Autodesk Fusion 360 part; units mm, degrees
note: some values were not read from the file. Set by a fixed rule: which sketch regions a step uses.
(part 2 of 4)
  spline S109 degree 3 poles (-112.0728, -32.2292) (-112.5404, -31.8601) (-113.2203, -31.6275) (-113.5837, -31.7122) knots 0 0 0 0 1 1 1 1
  spline S110 degree 3 poles (-136.2209, -38.6484) (-139.7578, -43.5067) (-144.003, -49.2146) (-147.0742, -52.9444) knots 0 0 0 0 1 1 1 1
  spline S111 degree 3 poles (-154.2165, -27.0184) (-154.4007, -27.683) (-154.551, -27.4601) (-154.6666, -26.3504) knots 0 0 0 0 1 1 1 1
  spline S112 degree 3 poles (-84.3741, -40.3079) (-87.8752, -40.018) (-88.8355, -39.1456) (-87.7319, -37.2577) knots 0 0 0 0 1 1 1 1
  spline S113 degree 3 poles (-140.3165, -99.6255) (-140.307, -99.0782) (-141.0618, -97.9071) (-141.9939, -97.0229) knots 0 0 0 0 1 1 1 1
  line L97 (-121.5387, -89.9657) -> (-118.5791, -90.609)
  spline S114 degree 3 poles (-154.7919, -33.624) (-155.1377, -31.5295) (-154.9908, -31.2048) (-153.5956, -30.9793) knots 0 0 0 0 1 1 1 1
  spline S115 degree 3 poles (-103.6508, -80.373) (-104.0694, -84.1491) (-102.7518, -86.3818) (-98.6044, -88.9248) knots 0 0 0 0 1 1 1 1
  spline S116 degree 3 poles (-104.4545, -159.4656) (-104.6393, -158.9576) (-105.2292, -158.3375) (-105.7651, -158.0876) knots 0 0 0 0 1 1 1 1
  line L98 (-76.19, -217.0111) -> (-79.4365, -211.2784)
  spline S117 degree 3 poles (-96.7029, -170.3232) (-100.0171, -162.0462) (-100.2006, -161.7333) (-102.1257, -161.073) knots 0 0 0 0 1 1 1 1
  spline S118 degree 3 poles (-106.4868, -123.3433) (-106.9706, -124.7012) (-107.6243, -126.5592) (-107.9395, -127.4722) knots 0 0 0 0 1 1 1 1
  line L99 (-151.1746, -82.8005) -> (-152.1113, -79.6578)
  spline S119 degree 3 poles (-164.6222, -35.8254) (-164.3798, -35.5183) (-164.0173, -35.7185) (-163.8165, -36.2701) knots 0 0 0 0 1 1 1 1
  spline S120 degree 3 poles (-97.3886, -94.7063) (-100.0855, -99.9855) (-102.1641, -106.0488) (-104.0281, -114.0757) knots 0 0 0 0 1 1 1 1
  spline S121 degree 3 poles (-116.5906, -88.5651) (-114.2332, -86.142) (-111.3799, -79.5261) (-109.9199, -73.0985) knots 0 0 0 0 1 1 1 1
  line L100 (-71.6837, -54.5973) -> (-71.6834, -54.5969)
  spline S122 degree 3 poles (-119.4232, -30.4738) (-125.5719, -30.4722) (-132.2129, -34.4961) (-136.2209, -38.6484) knots 0 0 0 0 1 1 1 1
  spline S123 degree 3 poles (-87.3826, -35.3672) (-87.8899, -33.9734) (-86.4389, -25.012) (-85.4231, -23.2654) knots 0 0 0 0 1 1 1 1
  spline S124 degree 3 poles (-154.6666, -26.3504) (-155.4003, -19.3112) (-156.3482, -18.6133) (-162.7786, -20.375) knots 0 0 0 0 1 1 1 1
  spline S125 degree 3 poles (-109.9199, -73.0985) (-108.891, -68.5684) (-108.2546, -67.383) (-107.6608, -68.8907) knots 0 0 0 0 1 1 1 1
  spline S126 degree 3 poles (-83.0888, -107.0535) (-83.9086, -107.766) (-83.3399, -110.3472) (-82.4356, -110.0181) knots 0 0 0 0 1 1 1 1
  spline S127 degree 3 poles (-145.3026, -92.1497) (-146.1903, -90.3535) (-147.6639, -88.2222) (-148.5772, -87.4136) knots 0 0 0 0 1 1 1 1
  line L101 (-127.616, -73.2152) -> (-127.616, -73.215)
  spline S128 degree 3 poles (-179.1592, -14.8194) (-179.6701, -15.4667) (-181.8024, -11.7834) (-183.7113, -6.9562) knots 0 0 0 0 1 1 1 1
  spline S129 degree 3 poles (-162.4907, -49.7556) (-162.586, -51.9164) (-162.5668, -52.4177) (-162.3525, -53.3552) knots 0 0 0 0 1 1 1 1
  spline S130 degree 3 poles (-108.3458, -30.6552) (-107.7548, -30.7777) (-107.7164, -30.5518) (-108.2282, -29.9629) knots 0 0 0 0 1 1 1 1
  spline S131 degree 3 poles (-107.3197, -33.1494) (-108.6187, -32.1334) (-109.3089, -30.4554) (-108.3458, -30.6552) knots 0 0 0 0 1 1 1 1
  spline S132 degree 3 poles (-130.5025, -128.6131) (-135.3605, -121.8502) (-135.4133, -121.7401) (-135.9917, -117.1824) knots 0 0 0 0 1 1 1 1
  spline S133 degree 3 poles (-82.4356, -110.0181) (-81.5449, -109.6939) (-77.0276, -113.218) (-76.5096, -114.6411) knots 0 0 0 0 1 1 1 1
  spline S134 degree 3 poles (-126.1453, -138.8187) (-126.7195, -138.8087) (-127.4424, -138.105) (-127.7519, -137.2548) knots 0 0 0 0 1 1 1 1
  spline S135 degree 3 poles (-139.0681, -102.1478) (-138.9659, -101.4044) (-139.1827, -100.8591) (-139.6164, -100.7692) knots 0 0 0 0 1 1 1 1
  line L102 (-95.4296, -90.8714) -> (-97.3886, -94.7063)
  spline S136 degree 3 poles (-108.2282, -29.9629) (-108.6756, -29.448) (-108.6885, -28.9597) (-108.2594, -28.7749) knots 0 0 0 0 1 1 1 1
  spline S137 degree 3 poles (-115.0249, -149.0253) (-116.7184, -147.2776) (-118.5469, -145.7771) (-120.0633, -144.8906) knots 0 0 0 0 1 1 1 1
  line L103 (-152.1113, -79.6578) -> (-148.5919, -78.2652)
  spline S138 degree 3 poles (-124.7918, -139.6875) (-124.9621, -139.2197) (-125.5712, -138.8287) (-126.1453, -138.8187) knots 0 0 0 0 1 1 1 1
  line L104 (-148.5919, -78.2652) -> (-145.0725, -76.8727)
  spline S139 degree 3 poles (-74.1947, -115.3174) (-73.0292, -114.8932) (-71.9308, -114.9941) (-71.1607, -115.5962) knots 0 0 0 0 1 1 1 1
  spline S140 degree 3 poles (-129.6791, -65.9357) (-125.8343, -62.6694) (-127.4522, -73.1016) (-127.616, -73.2152) knots 0 0 0 0 1 1 1 1
  spline S141 degree 3 poles (-93.212, -111.5023) (-91.5685, -106.4875) (-88.2032, -100.9795) (-84.6693, -97.5197) knots 0 0 0 0 1 1 1 1
  spline S142 degree 3 poles (-127.616, -73.215) (-127.919, -73.3253) (-128.2661, -73.1431) (-128.3872, -72.8102) knots 0 0 0 0 1 1 1 1
  spline S143 degree 3 poles (-137.8943, -108.0755) (-138.633, -105.4917) (-139.1612, -102.8242) (-139.0681, -102.1478) knots 0 0 0 0 1 1 1 1
  spline S144 degree 3 poles (-85.4231, -23.2654) (-84.2448, -21.2393) (-84.8036, -21.3276) (-87.2116, -23.5478) knots 0 0 0 0 1 1 1 1
  spline S145 degree 3 poles (-127.7519, -137.2548) (-128.1329, -136.2081) (-128.6652, -135.819) (-129.4007, -136.0498) knots 0 0 0 0 1 1 1 1
  spline S146 degree 3 poles (-133.2081, -68.992) (-131.2389, -68.4482) (-130.936, -67.0047) (-129.6791, -65.9357) knots 0 0 0 0 1 1 1 1
  spline S147 degree 3 poles (-183.7113, -6.9562) (-184.7798, -4.2542) (-185.4511, -3.3311) (-186.5872, -3.0015) knots 0 0 0 0 1 1 1 1
  spline S148 degree 3 poles (-103.4783, -30.4373) (-102.821, -31.518) (-102.6423, -32.3115) (-103.0249, -32.4507) knots 0 0 0 0 1 1 1 1
  line L105 (-118.5791, -90.609) -> (-116.5906, -88.5651)
  spline S149 degree 3 poles (-107.6608, -68.8907) (-107.497, -69.3066) (-106.4548, -71.4025) (-105.3449, -73.5484) knots 0 0 0 0 1 1 1 1
  spline S150 degree 3 poles (-103.1195, -33.1042) (-102.17, -33.8536) (-103.886, -34.7192) (-105.7404, -34.4262) knots 0 0 0 0 1 1 1 1
  spline S151 degree 3 poles (-165.6722, -35.9026) (-165.337, -36.1672) (-164.8645, -36.1324) (-164.6222, -35.8254) knots 0 0 0 0 1 1 1 1
  spline S152 degree 3 poles (-84.6693, -97.5197) (-83.6282, -96.5006) (-82.5684, -95.831) (-82.3142, -96.0317) knots 0 0 0 0 1 1 1 1
  spline S153 degree 3 poles (-148.5772, -87.4136) (-149.6517, -86.4623) (-150.5685, -84.8339) (-151.1746, -82.8005) knots 0 0 0 0 1 1 1 1
  spline S154 degree 3 poles (-104.0281, -114.0757) (-104.8966, -117.815) (-106.003, -121.9853) (-106.4868, -123.3433) knots 0 0 0 0 1 1 1 1
  spline S155 degree 3 poles (-95.9356, -117.5951) (-95.3387, -116.9936) (-94.113, -114.2518) (-93.212, -111.5023) knots 0 0 0 0 1 1 1 1
  spline S156 degree 3 poles (-165.5322, -47.9185) (-167.9275, -39.8001) (-167.9943, -34.07) (-165.6722, -35.9025) knots 0 0 0 0 1 1 1 1
  line L106 (-139.6588, -79.8807) -> (-139.6591, -79.8813)
  spline S157 degree 3 poles (-163.8165, -36.2701) (-163.3332, -37.5981) (-162.3816, -47.2782) (-162.4907, -49.7556) knots 0 0 0 0 1 1 1 1
  spline S158 degree 3 poles (-99.4834, -22.2152) (-102.7671, -24.1219) (-105.1902, -27.5695) (-103.4783, -30.4373) knots 0 0 0 0 1 1 1 1
  spline S159 degree 3 poles (-70.9678, -64.1804) (-71.0778, -65.837) (-71.2409, -67.2189) (-71.3304, -67.2515) knots 0 0 0 0 1 1 1 1
  spline S160 degree 3 poles (-100.1317, -132.8949) (-98.7815, -129.5666) (-97.5292, -125.0086) (-97.3489, -122.7659) knots 0 0 0 0 1 1 1 1
  spline S161 degree 3 poles (-113.5837, -31.7122) (-114.8758, -31.1202) (-118.9006, -30.5) (-119.4232, -30.4738) knots 0 0 0 0 1 1 1 1
  spline S162 degree 3 poles (-71.3304, -67.2515) (-72.5816, -66.2567) (-96.5427, -51.7484) (-92.0911, -45.0244) knots 0 0 0 0 1 1 1 1
  spline S163 degree 3 poles (-105.3449, -73.5484) (-103.5984, -76.9253) (-103.3705, -77.8432) (-103.6508, -80.373) knots 0 0 0 0 1 1 1 1
  spline S164 degree 3 poles (-87.7319, -37.2577) (-87.3803, -36.6562) (-87.2231, -35.8055) (-87.3826, -35.3672) knots 0 0 0 0 1 1 1 1
  spline S165 degree 3 poles (-147.0742, -52.9444) (-148.0276, -54.2206) (-148.1757, -54.2339) (-148.9598, -53.1145) knots 0 0 0 0 1 1 1 1
  spline S166 degree 3 poles (-97.3489, -122.7659) (-97.1686, -120.5233) (-96.5325, -118.1966) (-95.9356, -117.5951) knots 0 0 0 0 1 1 1 1
  line L107 (122.5483, 261.5188) -> (122.5506, 261.5232)
  spline S167 degree 3 poles (-177.1846, -17.5625) (-177.5438, -16.9549) (-178.0397, -15.9683) (-178.2865, -15.3701) knots 0 0 0 0 1 1 1 1
  spline S168 degree 3 poles (-110.1669, -137.8907) (-112.712, -151.3653) (-112.7265, -151.3976) (-115.0249, -149.0253) knots 0 0 0 0 1 1 1 1
  spline S169 degree 3 poles (-139.6164, -100.7692) (-140.0109, -100.6874) (-140.326, -100.1727) (-140.3165, -99.6255) knots 0 0 0 0 1 1 1 1
  line L108 (-165.6722, -35.9025) -> (-165.6722, -35.9026)
  spline S170 degree 3 poles (-91.5548, -189.9237) (-92.8333, -186.2605) (-93.4883, -183.3011) (-93.4037, -181.5704) knots 0 0 0 0 1 1 1 1
  spline S171 degree 3 poles (-105.7404, -34.4262) (-106.729, -34.2701) (-107.319, -34.0516) (-107.0516, -33.9408) knots 0 0 0 0 1 1 1 1
  spline S172 degree 3 poles (-84.6389, -203.663) (-86.6971, -201.6816) (-90.5134, -195.9478) (-89.9214, -195.7261) knots 0 0 0 0 1 1 1 1
  spline S173 degree 3 poles (-139.6591, -79.8813) (-136.6816, -81.5357) (-133.4883, -83.6932) (-132.5628, -84.676) knots 0 0 0 0 1 1 1 1
  spline S174 degree 3 poles (-173.3647, -20.7079) (-174.7646, -21.2174) (-175.2692, -20.8019) (-177.1846, -17.5625) knots 0 0 0 0 1 1 1 1
  spline S175 degree 3 poles (-107.9395, -127.4722) (-108.2547, -128.3851) (-109.2571, -133.0734) (-110.1669, -137.8907) knots 0 0 0 0 1 1 1 1
  spline S176 degree 3 poles (-169.6944, -20.9217) (-170.9251, -20.5173) (-172.5768, -20.4211) (-173.3647, -20.7079) knots 0 0 0 0 1 1 1 1
  spline S177 degree 3 poles (-105.7651, -158.0876) (-108.1851, -156.9591) (-106.086, -147.5724) (-100.1317, -132.8949) knots 0 0 0 0 1 1 1 1
  spline S178 degree 3 poles (-120.0633, -144.8906) (-120.7025, -144.5169) (-121.2171, -143.7303) (-121.2068, -143.1427) knots 0 0 0 0 1 1 1 1
  spline S179 degree 3 poles (-69.4601, -116.3603) (-69.1888, -116.2616) (-67.7713, -116.3006) (-66.31, -116.4471) knots 0 0 0 0 1 1 1 1
  spline S180 degree 3 poles (-141.9939, -97.0229) (-142.926, -96.1388) (-144.4149, -93.9458) (-145.3026, -92.1497) knots 0 0 0 0 1 1 1 1
  spline S181 degree 3 poles (-135.9917, -117.1824) (-136.2994, -114.7575) (-137.1556, -110.6593) (-137.8943, -108.0755) knots 0 0 0 0 1 1 1 1
  spline S182 degree 3 poles (-89.9214, -195.7261) (-89.7309, -195.6547) (-90.4659, -193.0438) (-91.5548, -189.9237) knots 0 0 0 0 1 1 1 1
  spline S183 degree 3 poles (-110.7717, -30.6482) (-111.1259, -32.417) (-111.4051, -32.7562) (-112.0728, -32.2292) knots 0 0 0 0 1 1 1 1
  line L109 (-98.6044, -88.9248) -> (-95.4296, -90.8714)
  spline S184 degree 3 poles (-108.9258, -28.4287) (-110.0298, -28.403) (-110.4149, -28.866) (-110.7717, -30.6482) knots 0 0 0 0 1 1 1 1
  spline S185 degree 3 poles (-53.9972, -105.1142) (-53.3719, -100.2884) (-56.959, -94.4448) (-60.8927, -93.8814) knots 0 0 0 0 1 1 1 1
  spline S186 degree 3 poles (-60.8927, -93.8814) (-63.6579, -93.4851) (-63.887, -92.6055) (-62.4815, -87.7805) knots 0 0 0 0 1 1 1 1
  spline S187 degree 3 poles (-162.3525, -53.3552) (-162.2722, -53.7063) (-162.5181, -54.107) (-162.8988, -54.2456) knots 0 0 0 0 1 1 1 1
  spline S188 degree 3 poles (-108.2594, -28.7749) (-107.8588, -28.6023) (-108.1586, -28.4465) (-108.9258, -28.4287) knots 0 0 0 0 1 1 1 1
  spline S189 degree 3 poles (-93.4037, -181.5704) (-93.2975, -179.3971) (-93.9219, -177.2686) (-96.7029, -170.3232) knots 0 0 0 0 1 1 1 1
  spline S190 degree 3 poles (-359.3827, -39.3133) (-362.0803, -44.2) (-364.097, -48.3222) (-363.8641, -48.4729) knots 0 0 0 0 1 1 1 1
  spline S191 degree 3 poles (-401.0815, -136.7584) (-401.0815, -135.2288) (-401.9958, -132.2563) (-403.1133, -130.1526) knots 0 0 0 0 1 1 1 1
  spline S192 degree 3 poles (-329.6558, -67.7504) (-332.7639, -68.9128) (-337.0362, -71.1394) (-339.1495, -72.6985) knots 0 0 0 0 1 1 1 1
  spline S193 degree 3 poles (-384.2382, -114.1572) (-389.3298, -115.1754) (-392.3756, -113.893) (-393.9618, -110.0632) knots 0 0 0 0 1 1 1 1
  spline S194 degree 3 poles (-407.6974, -152.4097) (-403.7766, -148.2524) (-399.8472, -144.8513) (-398.9647, -144.8513) knots 0 0 0 0 1 1 1 1
  line L110 (-359.0093, -106.5628) -> (-359.8673, -95.5242)
  spline S195 degree 3 poles (-322.8096, -64.7452) (-323.4669, -65.2358) (-326.5477, -66.5881) (-329.6558, -67.7504) knots 0 0 0 0 1 1 1 1
  spline S196 degree 3 poles (-354.4861, -55.414) (-354.4815, -55.8492) (-352.3092, -56.5716) (-349.6584, -57.0194) knots 0 0 0 0 1 1 1 1
  spline S197 degree 3 poles (-396.4605, -56.4196) (-395.926, -56.4196) (-394.7608, -54.2141) (-393.8711, -51.5183) knots 0 0 0 0 1 1 1 1
  spline S198 degree 3 poles (-398.9647, -144.8513) (-397.6998, -144.8513) (-397.754, -144.2899) (-399.2212, -142.1953) knots 0 0 0 0 1 1 1 1
  spline S199 degree 3 poles (-393.9618, -110.0632) (-395.9962, -105.1512) (-397.1166, -105.7296) (-398.5548, -112.4342) knots 0 0 0 0 1 1 1 1
  spline S200 degree 3 poles (-399.2212, -142.1953) (-400.2443, -140.7345) (-401.0815, -138.2879) (-401.0815, -136.7584) knots 0 0 0 0 1 1 1 1
  spline S201 degree 3 poles (-342.1423, -56.0668) (-340.6591, -55.095) (-334.9861, -52.7898) (-329.5358, -50.9442) knots 0 0 0 0 1 1 1 1
  spline S202 degree 3 poles (-393.1647, -142.443) (-391.8086, -142.443) (-383.16, -133.8081) (-383.1599, -132.4538) knots 0 0 0 0 1 1 1 1
  spline S203 degree 3 poles (-407.329, -91.376) (-407.9951, -90.5559) (-409.7681, -85.5329) (-411.269, -80.2141) knots 0 0 0 0 1 1 1 1
  spline S204 degree 3 poles (-393.318, -138.8579) (-393.7511, -140.8296) (-393.6821, -142.443) (-393.1647, -142.443) knots 0 0 0 0 1 1 1 1
  line L111 (-365.4073, -112.9997) -> (-359.0093, -106.5628)
  spline S205 degree 3 poles (-410.3748, -62.2295) (-409.1757, -61.4884) (-409.1713, -60.9969) (-410.3529, -59.8152) knots 0 0 0 0 1 1 1 1
  spline S206 degree 3 poles (-381.3187, -96.033) (-380.8394, -97.5683) (-379.913, -99.1676) (-379.2601, -99.5871) knots 0 0 0 0 1 1 1 1
  spline S207 degree 3 poles (-410.3529, -59.8152) (-412.3844, -57.7837) (-412.2152, -54.6361) (-409.9744, -52.7766) knots 0 0 0 0 1 1 1 1
  spline S208 degree 3 poles (-402.7721, -53.8254) (-399.8352, -55.2522) (-396.995, -56.4196) (-396.4605, -56.4196) knots 0 0 0 0 1 1 1 1
  spline S209 degree 3 poles (-379.2601, -99.5871) (-378.6072, -100.0066) (-378.4147, -100.9026) (-378.8323, -101.5782) knots 0 0 0 0 1 1 1 1
  spline S210 degree 3 poles (-350.5537, -99.6841) (-349.7543, -99.04) (-344.2602, -95.8368) (-338.345, -92.5656) knots 0 0 0 0 1 1 1 1
  line L112 (-322.8094, -64.7455) -> (-322.8096, -64.7452)
  spline S211 degree 3 poles (-379.6391, -94.6071) (-381.9765, -93.3561) (-382.1172, -93.4756) (-381.3187, -96.033) knots 0 0 0 0 1 1 1 1
  spline S212 degree 3 poles (-363.9321, -75.9411) (-355.8141, -72.1224) (-355.0753, -73.0985) (-355.0753, -87.6398) knots 0 0 0 0 1 1 1 1
  spline S213 degree 3 poles (-354.4778, -28.5764) (-354.4778, -29.5947) (-356.685, -34.4266) (-359.3827, -39.3133) knots 0 0 0 0 1 1 1 1
  spline S214 degree 3 poles (-349.6584, -57.0194) (-346.2683, -57.5922) (-344.0393, -57.3097) (-342.1423, -56.0668) knots 0 0 0 0 1 1 1 1
  spline S215 degree 3 poles (-433.5752, -170.9019) (-430.8685, -166.7624) (-423.3796, -161.6792) (-418.5714, -160.7174) knots 0 0 0 0 1 1 1 1
  spline S216 degree 3 poles (-313.2386, -75.6312) (-306.0084, -71.5505) (-305.2318, -69.4575) (-309.3317, -65.0938) knots 0 0 0 0 1 1 1 1
  spline S217 degree 3 poles (-238.2871, -16.6962) (-230.8144, -9.6389) (-227.6497, -7.419) (-217.2124, -1.9134) knots 0 0 0 0 1 1 1 1
  spline S218 degree 3 poles (-454.8506, -193.8468) (-449.9333, -190.6228) (-438.1872, -177.9547) (-433.5752, -170.9019) knots 0 0 0 0 1 1 1 1
  spline S219 degree 3 poles (-307.5734, -53.6039) (-304.1228, -53.4473) (-303.7162, -53.761) (-303.9287, -56.4153) knots 0 0 0 0 1 1 1 1
  spline S220 degree 3 poles (-393.8711, -51.5183) (-392.428, -47.1455) (-389.0192, -42.7421) (-384.1975, -39.0223) knots 0 0 0 0 1 1 1 1
  spline S221 degree 3 poles (-312.6717, -52.2447) (-312.0037, -51.8319) (-311.4572, -52.0085) (-311.4572, -52.6371) knots 0 0 0 0 1 1 1 1
  spline S222 degree 3 poles (-366.89, -16.9696) (-365.4879, -12.2211) (-356.7068, -0.0605) (-350.5917, 5.601) knots 0 0 0 0 1 1 1 1
  spline S223 degree 3 poles (-394.2901, -135.2727) (-392.9566, -135.2728) (-392.7212, -136.1411) (-393.318, -138.8579) knots 0 0 0 0 1 1 1 1
  spline S224 degree 3 poles (-418.5714, -160.7174) (-416.0694, -160.217) (-412.4596, -157.459) (-407.6974, -152.4097) knots 0 0 0 0 1 1 1 1
  spline S225 degree 3 poles (-378.354, -106.0615) (-376.8485, -110.0216) (-379.1088, -113.1312) (-384.2382, -114.1572) knots 0 0 0 0 1 1 1 1
  spline S226 degree 3 poles (-378.8323, -101.5782) (-379.2499, -102.2537) (-379.0346, -104.2713) (-378.354, -106.0615) knots 0 0 0 0 1 1 1 1
  spline S227 degree 3 poles (-398.5548, -112.4342) (-400.4467, -121.2546) (-397.8291, -135.2726) (-394.2901, -135.2727) knots 0 0 0 0 1 1 1 1
  spline S228 degree 3 poles (-342.5254, 15.9086) (-342.5254, 19.4558) (-332.7886, 21.3748) (-329.0332, 18.5679) knots 0 0 0 0 1 1 1 1
  spline S229 degree 3 poles (-403.1133, -130.1526) (-404.6599, -127.2412) (-405.2611, -122.3336) (-405.6314, -109.5978) knots 0 0 0 0 1 1 1 1
  spline S230 degree 3 poles (-365.0199, -66.3073) (-369.832, -61.6467) (-374.5603, -68.447) (-373.7194, -78.8195) knots 0 0 0 0 1 1 1 1
  spline S231 degree 3 poles (-383.1599, -132.4538) (-383.1599, -131.3301) (-377.9236, -125.5921) (-365.4073, -112.9997) knots 0 0 0 0 1 1 1 1
  spline S232 degree 3 poles (-350.5917, 5.601) (-348.7842, 7.2744) (-347.3054, 9.8682) (-347.3054, 11.3651) knots 0 0 0 0 1 1 1 1
  spline S233 degree 3 poles (-345.0961, -75.5333) (-347.5821, -75.5333) (-362.7421, -68.5136) (-365.0199, -66.3073) knots 0 0 0 0 1 1 1 1
  spline S234 degree 3 poles (-373.2522, -93.5142) (-376.3805, -95.519) (-377.5586, -95.7206) (-379.6391, -94.6071) knots 0 0 0 0 1 1 1 1
  spline S235 degree 3 poles (-303.9287, -56.4153) (-304.0603, -58.0584) (-303.8818, -61.4006) (-303.532, -63.8424) knots 0 0 0 0 1 1 1 1
  spline S236 degree 3 poles (-338.555, 3.701) (-340.4712, -0.1144) (-344.838, -8.5214) (-348.2586, -14.9809) knots 0 0 0 0 1 1 1 1
  spline S237 degree 3 poles (-348.2586, -14.9809) (-351.6792, -21.4404) (-354.4778, -27.5581) (-354.4778, -28.5764) knots 0 0 0 0 1 1 1 1
  spline S238 degree 3 poles (-347.3054, 11.3651) (-347.3054, 13.2899) (-346.6058, 14.0865) (-344.9154, 14.0865) knots 0 0 0 0 1 1 1 1
  spline S239 degree 3 poles (-323.6954, -82.9764) (-321.5535, -80.9736) (-316.8479, -77.6681) (-313.2386, -75.6312) knots 0 0 0 0 1 1 1 1
  spline S240 degree 3 poles (-316.8004, -63.0606) (-319.4481, -63.4967) (-322.1521, -64.2549) (-322.8094, -64.7455) knots 0 0 0 0 1 1 1 1
  spline S241 degree 3 poles (-329.5358, -50.9442) (-318.8808, -47.3363) (-315.9974, -47.6815) (-315.2579, -52.6535) knots 0 0 0 0 1 1 1 1
  spline S242 degree 3 poles (-363.8641, -48.4729) (-356.973, -52.9332) (-354.4925, -54.769) (-354.4861, -55.414) knots 0 0 0 0 1 1 1 1
  spline S243 degree 3 poles (-309.3317, -65.0938) (-311.5923, -62.6875) (-312.7018, -62.3855) (-316.8004, -63.0606) knots 0 0 0 0 1 1 1 1
  spline S244 degree 3 poles (-315.2579, -52.6535) (-315.0479, -54.0652) (-314.344, -55.2202) (-313.6936, -55.2202) knots 0 0 0 0 1 1 1 1
  spline S245 degree 3 poles (-313.1987, -54.1078) (-313.5769, -53.4959) (-313.3397, -52.6576) (-312.6717, -52.2447) knots 0 0 0 0 1 1 1 1
  spline S246 degree 3 poles (-247.1739, -30.0848) (-244.6533, -29.9662) (-241.1428, -25.4651) (-241.7525, -23.1333) knots 0 0 0 0 1 1 1 1
  spline S247 degree 3 poles (-313.6936, -55.2202) (-313.0432, -55.2202) (-312.8205, -54.7196) (-313.1987, -54.1078) knots 0 0 0 0 1 1 1 1
  spline S248 degree 3 poles (-409.9744, -52.7766) (-408.4269, -51.4923) (-407.2094, -51.6696) (-402.7721, -53.8254) knots 0 0 0 0 1 1 1 1
  line L113 (-364.04, -85.2611) -> (-364.0385, -85.26)
  spline S249 degree 3 poles (-361.2702, -83.5702) (-361.9723, -82.3901) (-364.04, -83.6524) (-364.04, -85.2611) knots 0 0 0 0 1 1 1 1
  spline S250 degree 3 poles (-369.8141, -79.4171) (-369.595, -78.9241) (-366.9481, -77.36) (-363.9321, -75.9411) knots 0 0 0 0 1 1 1 1
  spline S251 degree 3 poles (-411.269, -80.2141) (-414.078, -70.2597) (-413.7834, -64.3357) (-410.3748, -62.2295) knots 0 0 0 0 1 1 1 1
  spline S252 degree 3 poles (-339.1495, -72.6985) (-341.2628, -74.2576) (-343.9388, -75.5333) (-345.0961, -75.5333) knots 0 0 0 0 1 1 1 1
  spline S253 degree 3 poles (-373.7194, -78.8195) (-373.5893, -80.4246) (-370.4737, -80.9013) (-369.8141, -79.4171) knots 0 0 0 0 1 1 1 1
  spline S254 degree 3 poles (-294.9276, -62.3044) (-290.5449, -59.0168) (-282.9288, -53.2546) (-278.0022, -49.4997) knots 0 0 0 0 1 1 1 1
  spline S255 degree 3 poles (-405.6314, -109.5978) (-405.899, -100.3959) (-406.6629, -92.1961) (-407.329, -91.376) knots 0 0 0 0 1 1 1 1
  spline S256 degree 3 poles (-241.7525, -23.1333) (-242.2366, -21.2822) (-241.2992, -19.5409) (-238.2871, -16.6962) knots 0 0 0 0 1 1 1 1
  spline S257 degree 3 poles (-359.8673, -95.5242) (-360.3392, -89.4533) (-360.9705, -84.0738) (-361.2702, -83.5702) knots 0 0 0 0 1 1 1 1
  spline S258 degree 3 poles (-355.0753, -87.6398) (-355.0753, -99.9681) (-354.1072, -102.5467) (-350.5537, -99.6841) knots 0 0 0 0 1 1 1 1
  spline S259 degree 3 poles (-364.0385, -85.26) (-364.0385, -86.6747) (-367.7052, -89.9597) (-373.2522, -93.5142) knots 0 0 0 0 1 1 1 1
  spline S260 degree 3 poles (-329.0355, 18.5722) (-326.7611, 16.8724) (-327.4338, 15.4917) (-331.9278, 12.6358) knots 0 0 0 0 1 1 1 1
  line L114 (-303.532, -63.8424) -> (-302.8961, -68.2819)
  spline S261 degree 3 poles (-278.0022, -49.4997) (-269.6477, -43.1315) (-249.0728, -30.1745) (-247.1739, -30.0848) knots 0 0 0 0 1 1 1 1
  spline S262 degree 3 poles (-331.9278, 12.6358) (-333.6565, 11.5373) (-336.6388, 7.5165) (-338.555, 3.701) knots 0 0 0 0 1 1 1 1
  spline S263 degree 3 poles (-344.9154, 14.0865) (-343.5703, 14.0865) (-342.5254, 14.8832) (-342.5254, 15.9086) knots 0 0 0 0 1 1 1 1
  spline S264 degree 3 poles (-338.345, -92.5656) (-332.4297, -89.2945) (-325.8373, -84.9793) (-323.6954, -82.9764) knots 0 0 0 0 1 1 1 1
  line L115 (-217.2124, -1.9134) -> (-213.5849, 0)
  spline S265 degree 3 poles (-311.4572, -52.6371) (-311.4572, -53.2657) (-309.7095, -53.7008) (-307.5734, -53.6039) knots 0 0 0 0 1 1 1 1
  line L116 (-302.8961, -68.2819) -> (-294.9276, -62.3044)
  spline S266 degree 3 poles (-384.1975, -39.0223) (-379.0998, -35.0894) (-368.1026, -21.0773) (-366.89, -16.9696) knots 0 0 0 0 1 1 1 1
  spline S267 degree 3 poles (-469.9, -207.2338) (-460.9906, -198.8048) (-456.9343, -195.2125) (-454.8506, -193.8468) knots 0.162411 0.162411 0.162411 0.162411 1 1 1 1
  spline S268 degree 3 poles (-469.9, -207.2338) (-460.9906, -198.8048) (-456.9343, -195.2125) (-454.8506, -193.8468) knots 0.162411 0.162411 0.162411 0.162411 1 1 1 1
  line L117 (-340.44, 0) -> (-355.8194, 0)
  line L118 (-189.0051, 0) -> (-213.5849, 0)
  line L119 (-76.19, -217.0111) -> (-469.9, -215.9)
  line L120 (-469.9, -215.9) -> (-469.9, -207.2338)
  constraint coincident L85 L95.end
  constraint coincident L85 L90.end
  constraint coincident L86 S267.start
  constraint coincident S236 L117.start
  constraint coincident L85 L117.start
  constraint coincident S41 L117.end
  constraint coincident L86.end L87.start
extrude "Extrude2" add sketch "Sketch2" along normal blind 12.7 contours L85 L86 L87 S2 S3 S4 S5 S6 S7 S8 S9 S10 S11 S12 S13 S14 S15 S16 S17 L88 L89 S18 S19 S20 S21 S22 L90 S23 S24 S25 S26 S27 S28 S29 S30 S31 S32 S33 S34 S35 S36 S37 S38 S39 S40 S41 S78 S79 S81 S82 S84 S85 L95 S86 S88 S89 S90 S92 S94 S96 S97 S99 S100 S102 S103 S105 S106 S108 S109 S110 S111 S112 S114 S116 L98 S117 S122 S123 S124 S126 S128 S130 S131 S133 S136 S139 S141 S144 S147 S148 S150 S152 S155 S158 S160 S161 S164 S165 S166 S167 S170 S171 S172 S174 S176 S177 S179 S182 S183 S184 S185 S186 S188 S189 S190 S191 S194 S196 S197 S198 S200 S201 S203 S205 S207 S208 S213 S214 S215 S217 S218 S219 S220 S221 S222 S224 S229 S235 S236 S237 S241 S242 S244 S245 S246 S247 S248 S251 S254 S255 S256 L114 S261 L115 S265 L116 S266 S267 S268 L117 L118 L120 bodies 1
sketch "Sketch3" plane through (0, 0, 38.1) normal (0, 0, 1) x (-1, 0, 0)
  spline S0 degree 3 poles (-373.2522, -93.5142) (-367.7052, -89.9597) (-364.0385, -86.6747) (-364.0385, -85.26) knots -1 -1 -1 -1 0 0 0 0
  line L0 (-364.0385, -85.26) -> (-364.04, -85.2611)
  spline S1 degree 3 poles (-364.04, -85.2611) (-364.04, -83.6524) (-361.9723, -82.3901) (-361.2702, -83.5702) knots -1 -1 -1 -1 0 0 0 0
  spline S2 degree 3 poles (-361.2702, -83.5702) (-360.9705, -84.0738) (-360.3392, -89.4533) (-359.8673, -95.5242) knots -1 -1 -1 -1 0 0 0 0
  line L1 (-359.8673, -95.5242) -> (-359.0093, -106.5628)
  line L2 (-359.0093, -106.5628) -> (-365.4073, -112.9997)
  spline S3 degree 3 poles (-365.4073, -112.9997) (-377.9236, -125.5921) (-383.1599, -131.3301) (-383.1599, -132.4538) knots -1 -1 -1 -1 0 0 0 0
  spline S4 degree 3 poles (-383.1599, -132.4538) (-383.16, -133.8081) (-391.8086, -142.443) (-393.1647, -142.443) knots -1 -1 -1 -1 0 0 0 0
  spline S5 degree 3 poles (-393.1647, -142.443) (-393.6821, -142.443) (-393.7511, -140.8296) (-393.318, -138.8579) knots -1 -1 -1 -1 0 0 0 0
  spline S6 degree 3 poles (-393.318, -138.8579) (-392.7212, -136.1411) (-392.9566, -135.2728) (-394.2901, -135.2727) knots -1 -1 -1 -1 0 0 0 0
  spline S7 degree 3 poles (-394.2901, -135.2727) (-397.8291, -135.2726) (-400.4467, -121.2546) (-398.5548, -112.4342) knots -1 -1 -1 -1 0 0 0 0
  spline S8 degree 3 poles (-398.5548, -112.4342) (-397.1166, -105.7296) (-395.9962, -105.1512) (-393.9618, -110.0632) knots -1 -1 -1 -1 0 0 0 0
  spline S9 degree 3 poles (-393.9618, -110.0632) (-392.3756, -113.893) (-389.3298, -115.1754) (-384.2382, -114.1572) knots -1 -1 -1 -1 0 0 0 0
  spline S10 degree 3 poles (-384.2382, -114.1572) (-379.1088, -113.1312) (-376.8485, -110.0216) (-378.354, -106.0615) knots -1 -1 -1 -1 0 0 0 0
  spline S11 degree 3 poles (-378.354, -106.0615) (-379.0346, -104.2713) (-379.2499, -102.2537) (-378.8323, -101.5782) knots -1 -1 -1 -1 0 0 0 0
  spline S12 degree 3 poles (-378.8323, -101.5782) (-378.4147, -100.9026) (-378.6072, -100.0066) (-379.2601, -99.5871) knots -1 -1 -1 -1 0 0 0 0
  spline S13 degree 3 poles (-379.2601, -99.5871) (-379.913, -99.1676) (-380.8394, -97.5683) (-381.3187, -96.033) knots -1 -1 -1 -1 0 0 0 0
  spline S14 degree 3 poles (-381.3187, -96.033) (-382.1172, -93.4756) (-381.9765, -93.3561) (-379.6391, -94.6071) knots -1 -1 -1 -1 0 0 0 0
  spline S15 degree 3 poles (-379.6391, -94.6071) (-377.5586, -95.7206) (-376.3805, -95.519) (-373.2522, -93.5142) knots -1 -1 -1 -1 0 0 0 0
  circle A0 centre (-444.5, -190.5) radius 4.1275
  circle A1 centre (-234.95, -107.95) radius 3.175
  arc A2 (-251.0881, -136.2619) -> (-249.292, -136.2619) centre (-250.19, -135.3638) ccw
  line L3 (-251.0881, -136.2619) -> (-253.628, -133.7219)
  arc A3 (-254, -132.8239) -> (-253.628, -133.7219) centre (-252.73, -132.8239) ccw
  line L4 (-254, -132.8239) -> (-254, -113.5561)
  arc A4 (-253.628, -112.658) -> (-254, -113.5561) centre (-252.73, -113.5561) ccw
  line L5 (-253.628, -112.658) -> (-251.088, -110.118)
  arc A5 (-249.292, -110.118) -> (-251.088, -110.118) centre (-250.19, -111.0161) ccw
  line L6 (-249.292, -110.118) -> (-246.752, -112.658)
  arc A6 (-246.38, -113.556) -> (-246.752, -112.658) centre (-247.65, -113.556) ccw
  line L7 (-246.38, -113.556) -> (-246.38, -132.8238)
  arc A7 (-246.752, -133.7219) -> (-246.38, -132.8238) centre (-247.65, -132.8238) ccw
  line L8 (-246.752, -133.7219) -> (-249.292, -136.2619)
  arc A8 (-275.962, -107.052) -> (-275.962, -108.848) centre (-275.0639, -107.95) ccw
  line L9 (-275.962, -107.052) -> (-273.422, -104.512)
  arc A9 (-272.5239, -104.14) -> (-273.422, -104.512) centre (-272.5239, -105.41) ccw
  line L10 (-272.5239, -104.14) -> (-255.796, -104.14)
  arc A10 (-254.898, -104.512) -> (-255.796, -104.14) centre (-255.796, -105.41) ccw
  line L11 (-254.898, -104.512) -> (-252.358, -107.052)
  arc A11 (-252.358, -108.848) -> (-252.358, -107.052) centre (-253.256, -107.95) ccw
  line L12 (-252.358, -108.848) -> (-254.898, -111.388)
  arc A12 (-255.796, -111.76) -> (-254.898, -111.388) centre (-255.796, -110.49) ccw
  line L13 (-255.796, -111.76) -> (-272.5239, -111.76)
  arc A13 (-273.422, -111.388) -> (-272.5239, -111.76) centre (-272.5239, -110.49) ccw
  line L14 (-273.422, -111.388) -> (-275.962, -108.848)
  arc A14 (-255.796, -172.72) -> (-254.898, -172.348) centre (-255.796, -171.45) ccw
  line L15 (-255.796, -172.72) -> (-272.5239, -172.72)
  arc A15 (-273.422, -172.348) -> (-272.5239, -172.72) centre (-272.5239, -171.45) ccw
  line L16 (-273.422, -172.348) -> (-275.962, -169.808)
  arc A16 (-275.962, -168.012) -> (-275.962, -169.808) centre (-275.0639, -168.91) ccw
  line L17 (-275.962, -168.012) -> (-273.422, -165.472)
  arc A17 (-272.5239, -165.1) -> (-273.422, -165.472) centre (-272.5239, -166.37) ccw
  line L18 (-272.5239, -165.1) -> (-255.796, -165.1)
  arc A18 (-254.898, -165.472) -> (-255.796, -165.1) centre (-255.796, -166.37) ccw
  line L19 (-254.898, -165.472) -> (-252.358, -168.012)
  arc A19 (-252.358, -169.808) -> (-252.358, -168.012) centre (-253.256, -168.91) ccw
  line L20 (-252.358, -169.808) -> (-254.898, -172.348)
  arc A20 (-217.542, -137.532) -> (-217.542, -139.328) centre (-216.644, -138.43) ccw
  line L21 (-217.542, -137.532) -> (-215.002, -134.992)
  arc A21 (-214.104, -134.62) -> (-215.002, -134.992) centre (-214.104, -135.89) ccw
  line L22 (-214.104, -134.62) -> (-197.3761, -134.62)
  arc A22 (-196.478, -134.992) -> (-197.3761, -134.62) centre (-197.3761, -135.89) ccw
  line L23 (-196.478, -134.992) -> (-193.938, -137.532)
  arc A23 (-193.938, -139.328) -> (-193.938, -137.532) centre (-194.8361, -138.43) ccw
  line L24 (-193.938, -139.328) -> (-196.478, -141.868)
  arc A24 (-197.3761, -142.24) -> (-196.478, -141.868) centre (-197.3761, -140.97) ccw
  line L25 (-197.3761, -142.24) -> (-214.104, -142.24)
  arc A25 (-215.002, -141.868) -> (-214.104, -142.24) centre (-214.104, -140.97) ccw
  line L26 (-215.002, -141.868) -> (-217.542, -139.328)
  arc A26 (-216.272, -164.202) -> (-215.9, -163.3039) centre (-217.17, -163.3039) ccw
  line L27 (-216.272, -164.202) -> (-218.812, -166.742)
  arc A27 (-220.608, -166.742) -> (-218.812, -166.742) centre (-219.71, -165.8439) ccw
  line L28 (-220.608, -166.742) -> (-223.148, -164.202)
  arc A28 (-223.52, -163.304) -> (-223.148, -164.202) centre (-222.25, -163.304) ccw
  line L29 (-223.52, -163.304) -> (-223.52, -144.0362)
  arc A29 (-223.148, -143.1381) -> (-223.52, -144.0362) centre (-222.25, -144.0362) ccw
  line L30 (-223.148, -143.1381) -> (-220.608, -140.5981)
  arc A30 (-218.8119, -140.5981) -> (-220.608, -140.5981) centre (-219.71, -141.4962) ccw
  line L31 (-218.8119, -140.5981) -> (-216.272, -143.1381)
  arc A31 (-215.9, -144.0361) -> (-216.272, -143.1381) centre (-217.17, -144.0361) ccw
  line L32 (-215.9, -144.0361) -> (-215.9, -163.3039)
  arc A32 (-193.938, -169.808) -> (-193.938, -168.012) centre (-194.8361, -168.91) ccw
  line L33 (-193.938, -169.808) -> (-196.478, -172.348)
  arc A33 (-197.3761, -172.72) -> (-196.478, -172.348) centre (-197.3761, -171.45) ccw
  line L34 (-197.3761, -172.72) -> (-214.104, -172.72)
  arc A34 (-215.002, -172.348) -> (-214.104, -172.72) centre (-214.104, -171.45) ccw
  line L35 (-215.002, -172.348) -> (-217.542, -169.808)
  arc A35 (-217.542, -168.012) -> (-217.542, -169.808) centre (-216.644, -168.91) ccw
  line L36 (-217.542, -168.012) -> (-215.002, -165.472)
  arc A36 (-214.104, -165.1) -> (-215.002, -165.472) centre (-214.104, -166.37) ccw
  line L37 (-214.104, -165.1) -> (-197.3761, -165.1)
  arc A37 (-196.478, -165.472) -> (-197.3761, -165.1) centre (-197.3761, -166.37) ccw
  line L38 (-196.478, -165.472) -> (-193.938, -168.012)
  arc A38 (-251.088, -166.742) -> (-249.292, -166.742) centre (-250.19, -165.8439) ccw
  line L39 (-251.088, -166.742) -> (-253.628, -164.202)
  arc A39 (-254, -163.3039) -> (-253.628, -164.202) centre (-252.73, -163.3039) ccw
  line L40 (-254, -163.3039) -> (-254, -144.0361)
  arc A40 (-253.628, -143.1381) -> (-254, -144.0361) centre (-252.73, -144.0361) ccw
  line L41 (-253.628, -143.1381) -> (-251.0881, -140.5981)
  arc A41 (-249.292, -140.5981) -> (-251.0881, -140.5981) centre (-250.19, -141.4962) ccw
  line L42 (-249.292, -140.5981) -> (-246.752, -143.1381)
  arc A42 (-246.38, -144.0362) -> (-246.752, -143.1381) centre (-247.65, -144.0362) ccw
  line L43 (-246.38, -144.0362) -> (-246.38, -163.304)
  arc A43 (-246.752, -164.202) -> (-246.38, -163.304) centre (-247.65, -163.304) ccw
  line L44 (-246.752, -164.202) -> (-249.292, -166.742)
  arc A44 (-281.94, -132.824) -> (-281.568, -133.722) centre (-280.67, -132.824) ccw
  line L45 (-281.94, -132.824) -> (-281.94, -113.5561)
  arc A45 (-281.568, -112.658) -> (-281.94, -113.5561) centre (-280.67, -113.5561) ccw
  line L46 (-281.568, -112.658) -> (-279.028, -110.118)
  arc A46 (-277.232, -110.118) -> (-279.028, -110.118) centre (-278.13, -111.016) ccw
  line L47 (-277.232, -110.118) -> (-274.692, -112.658)
  arc A47 (-274.32, -113.5561) -> (-274.692, -112.658) centre (-275.59, -113.5561) ccw
  line L48 (-274.32, -113.5561) -> (-274.32, -132.824)
  arc A48 (-274.692, -133.722) -> (-274.32, -132.824) centre (-275.59, -132.824) ccw
  line L49 (-274.692, -133.722) -> (-277.232, -136.262)
  arc A49 (-279.028, -136.262) -> (-277.232, -136.262) centre (-278.13, -135.364) ccw
  line L50 (-279.028, -136.262) -> (-281.568, -133.722)
  arc A50 (-195.58, -163.3039) -> (-195.208, -164.202) centre (-194.31, -163.3039) ccw
  line L51 (-195.58, -163.3039) -> (-195.58, -144.036)
  arc A51 (-195.208, -143.138) -> (-195.58, -144.036) centre (-194.31, -144.036) ccw
  line L52 (-195.208, -143.138) -> (-192.668, -140.598)
  arc A52 (-190.872, -140.598) -> (-192.668, -140.598) centre (-191.77, -141.496) ccw
  line L53 (-190.872, -140.598) -> (-188.332, -143.138)
  arc A53 (-187.96, -144.036) -> (-188.332, -143.138) centre (-189.23, -144.036) ccw
  line L54 (-187.96, -144.036) -> (-187.96, -163.3039)
  arc A54 (-188.332, -164.202) -> (-187.96, -163.3039) centre (-189.23, -163.3039) ccw
  line L55 (-188.332, -164.202) -> (-190.872, -166.742)
  arc A55 (-192.668, -166.742) -> (-190.872, -166.742) centre (-191.77, -165.844) ccw
  line L56 (-192.668, -166.742) -> (-195.208, -164.202)
  circle A56 centre (-457.2, -203.2) radius 0.635
  arc A57 (-273.422, -141.868) -> (-272.5239, -142.24) centre (-272.5239, -140.97) ccw
  line L57 (-273.422, -141.868) -> (-275.962, -139.328)
  arc A58 (-275.962, -137.532) -> (-275.962, -139.328) centre (-275.0639, -138.43) ccw
  line L58 (-275.962, -137.532) -> (-273.422, -134.992)
  arc A59 (-272.5239, -134.62) -> (-273.422, -134.992) centre (-272.5239, -135.89) ccw
  line L59 (-272.5239, -134.62) -> (-255.796, -134.62)
  arc A60 (-254.898, -134.992) -> (-255.796, -134.62) centre (-255.796, -135.89) ccw
  line L60 (-254.898, -134.992) -> (-252.358, -137.532)
  arc A61 (-252.358, -139.328) -> (-252.358, -137.532) centre (-253.256, -138.43) ccw
  line L61 (-252.358, -139.328) -> (-254.898, -141.868)
  arc A62 (-255.796, -142.24) -> (-254.898, -141.868) centre (-255.796, -140.97) ccw
  line L62 (-255.796, -142.24) -> (-272.5239, -142.24)
  arc A63 (-274.32, -144.036) -> (-274.692, -143.138) centre (-275.59, -144.036) ccw
  line L63 (-274.32, -144.036) -> (-274.32, -163.3039)
  arc A64 (-274.692, -164.202) -> (-274.32, -163.3039) centre (-275.59, -163.3039) ccw
  line L64 (-274.692, -164.202) -> (-277.232, -166.742)
  arc A65 (-279.028, -166.742) -> (-277.232, -166.742) centre (-278.13, -165.844) ccw
  line L65 (-279.028, -166.742) -> (-281.568, -164.202)
  arc A66 (-281.94, -163.3039) -> (-281.568, -164.202) centre (-280.67, -163.3039) ccw
  line L66 (-281.94, -163.3039) -> (-281.94, -144.036)
  arc A67 (-281.568, -143.138) -> (-281.94, -144.036) centre (-280.67, -144.036) ccw
  line L67 (-281.568, -143.138) -> (-279.028, -140.598)
  arc A68 (-277.232, -140.598) -> (-279.028, -140.598) centre (-278.13, -141.496) ccw
  line L68 (-277.232, -140.598) -> (-274.692, -143.138)
  arc A69 (-215.002, -111.388) -> (-214.104, -111.76) centre (-214.104, -110.49) ccw
  line L69 (-215.002, -111.388) -> (-217.542, -108.848)
  arc A70 (-217.542, -107.052) -> (-217.542, -108.848) centre (-216.644, -107.95) ccw
  line L70 (-217.542, -107.052) -> (-215.002, -104.512)
  arc A71 (-214.104, -104.14) -> (-215.002, -104.512) centre (-214.104, -105.41) ccw
  line L71 (-214.104, -104.14) -> (-197.3761, -104.14)
  arc A72 (-196.478, -104.512) -> (-197.3761, -104.14) centre (-197.3761, -105.41) ccw
  line L72 (-196.478, -104.512) -> (-193.938, -107.052)
  arc A73 (-193.938, -108.848) -> (-193.938, -107.052) centre (-194.8361, -107.95) ccw
  line L73 (-193.938, -108.848) -> (-196.478, -111.388)
  arc A74 (-197.3761, -111.76) -> (-196.478, -111.388) centre (-197.3761, -110.49) ccw
  line L74 (-197.3761, -111.76) -> (-214.104, -111.76)
  arc A75 (-216.272, -133.7219) -> (-215.9, -132.8239) centre (-217.17, -132.8239) ccw
  line L75 (-216.272, -133.7219) -> (-218.8119, -136.2619)
  arc A76 (-220.608, -136.2619) -> (-218.8119, -136.2619) centre (-219.71, -135.3638) ccw
  line L76 (-220.608, -136.2619) -> (-223.148, -133.7219)
  arc A77 (-223.52, -132.8238) -> (-223.148, -133.7219) centre (-222.25, -132.8238) ccw
  line L77 (-223.52, -132.8238) -> (-223.52, -113.556)
  arc A78 (-223.148, -112.658) -> (-223.52, -113.556) centre (-222.25, -113.556) ccw
  line L78 (-223.148, -112.658) -> (-220.608, -110.118)
  arc A79 (-218.812, -110.118) -> (-220.608, -110.118) centre (-219.71, -111.0161) ccw
  line L79 (-218.812, -110.118) -> (-216.272, -112.658)
  arc A80 (-215.9, -113.5561) -> (-216.272, -112.658) centre (-217.17, -113.5561) ccw
  line L80 (-215.9, -113.5561) -> (-215.9, -132.8239)
  arc A81 (-195.58, -132.824) -> (-195.208, -133.722) centre (-194.31, -132.824) ccw
  line L81 (-195.58, -132.824) -> (-195.58, -113.5561)
  arc A82 (-195.208, -112.658) -> (-195.58, -113.5561) centre (-194.31, -113.5561) ccw
  line L82 (-195.208, -112.658) -> (-192.668, -110.118)
  arc A83 (-190.872, -110.118) -> (-192.668, -110.118) centre (-191.77, -111.016) ccw
  line L83 (-190.872, -110.118) -> (-188.332, -112.658)
  arc A84 (-187.96, -113.5561) -> (-188.332, -112.658) centre (-189.23, -113.5561) ccw
  line L84 (-187.96, -113.5561) -> (-187.96, -132.824)
  arc A85 (-188.332, -133.722) -> (-187.96, -132.824) centre (-189.23, -132.824) ccw
  line L85 (-188.332, -133.722) -> (-190.872, -136.262)
  arc A86 (-192.668, -136.262) -> (-190.872, -136.262) centre (-191.77, -135.364) ccw
  line L86 (-192.668, -136.262) -> (-195.208, -133.722)
  spline S16 degree 3 poles (-70.9678, -64.1804) (-71.0778, -65.837) (-71.2409, -67.2189) (-71.3304, -67.2515) knots 0 0 0 0 1 1 1 1
  spline S17 degree 3 poles (-71.3304, -67.2515) (-72.5816, -66.2567) (-96.5427, -51.7484) (-92.0911, -45.0244) knots 0 0 0 0 1 1 1 1
  spline S18 degree 3 poles (-92.0911, -45.0244) (-85.2571, -44.0629) (-76.1399, -51.6985) (-71.6837, -54.5973) knots 0 0 0 0 1 1 1 1
  line L87 (-71.6837, -54.5973) -> (-71.6834, -54.5969)
  spline S19 degree 3 poles (-71.6834, -54.5969) (-69.8327, -55.7835) (-69.5192, -56.239) (-69.9128, -57.1685) knots 0 0 0 0 1 1 1 1
  spline S20 degree 3 poles (-69.9128, -57.1685) (-70.176, -57.7898) (-70.3353, -58.7343) (-70.2669, -59.2672) knots 0 0 0 0 1 1 1 1
  spline S21 degree 3 poles (-70.2669, -59.2672) (-70.3926, -60.9836) (-70.8659, -62.7082) (-70.9678, -64.1804) knots 0 0 0 0 1 1 1 1
  spline S22 degree 3 poles (-162.4907, -49.7556) (-162.586, -51.9164) (-162.5668, -52.4177) (-162.3525, -53.3552) knots 0 0 0 0 1 1 1 1
  spline S23 degree 3 poles (-162.3525, -53.3552) (-162.2722, -53.7063) (-162.5181, -54.107) (-162.8988, -54.2456) knots 0 0 0 0 1 1 1 1
  spline S24 degree 3 poles (-162.8988, -54.2456) (-163.3963, -54.4266) (-164.1374, -52.646) (-165.5322, -47.9185) knots 0 0 0 0 1 1 1 1
  spline S25 degree 3 poles (-165.5322, -47.9185) (-167.9275, -39.8001) (-167.9943, -34.07) (-165.6722, -35.9025) knots 0 0 0 0 1 1 1 1
  line L88 (-165.6722, -35.9025) -> (-165.6722, -35.9026)
  spline S26 degree 3 poles (-165.6722, -35.9026) (-165.337, -36.1672) (-164.8645, -36.1324) (-164.6222, -35.8254) knots 0 0 0 0 1 1 1 1
  spline S27 degree 3 poles (-164.6222, -35.8254) (-164.3798, -35.5183) (-164.0173, -35.7185) (-163.8165, -36.2701) knots 0 0 0 0 1 1 1 1
  spline S28 degree 3 poles (-163.8165, -36.2701) (-163.3332, -37.5981) (-162.3816, -47.2782) (-162.4907, -49.7556) knots 0 0 0 0 1 1 1 1
  spline S29 degree 3 poles (-103.6508, -80.373) (-104.0694, -84.1491) (-102.7518, -86.3818) (-98.6044, -88.9248) knots 0 0 0 0 1 1 1 1
  line L89 (-98.6044, -88.9248) -> (-95.4296, -90.8714)
  line L90 (-95.4296, -90.8714) -> (-97.3886, -94.7063)
  spline S30 degree 3 poles (-97.3886, -94.7063) (-100.0855, -99.9855) (-102.1641, -106.0488) (-104.0281, -114.0757) knots 0 0 0 0 1 1 1 1
  spline S31 degree 3 poles (-104.0281, -114.0757) (-104.8966, -117.815) (-106.003, -121.9853) (-106.4868, -123.3433) knots 0 0 0 0 1 1 1 1
  spline S32 degree 3 poles (-106.4868, -123.3433) (-106.9706, -124.7012) (-107.6243, -126.5592) (-107.9395, -127.4722) knots 0 0 0 0 1 1 1 1
  spline S33 degree 3 poles (-107.9395, -127.4722) (-108.2547, -128.3851) (-109.2571, -133.0734) (-110.1669, -137.8907) knots 0 0 0 0 1 1 1 1
  spline S34 degree 3 poles (-110.1669, -137.8907) (-112.712, -151.3653) (-112.7265, -151.3976) (-115.0249, -149.0253) knots 0 0 0 0 1 1 1 1
  spline S35 degree 3 poles (-115.0249, -149.0253) (-116.7184, -147.2776) (-118.5469, -145.7771) (-120.0633, -144.8906) knots 0 0 0 0 1 1 1 1
  spline S36 degree 3 poles (-120.0633, -144.8906) (-120.7025, -144.5169) (-121.2171, -143.7303) (-121.2068, -143.1427) knots 0 0 0 0 1 1 1 1
  spline S37 degree 3 poles (-121.2068, -143.1427) (-121.1966, -142.549) (-121.9202, -141.7328) (-122.8353, -141.3061) knots 0 0 0 0 1 1 1 1
  spline S38 degree 3 poles (-122.8353, -141.3061) (-123.7411, -140.8837) (-124.6215, -140.1553) (-124.7918, -139.6875) knots 0 0 0 0 1 1 1 1
  spline S39 degree 3 poles (-124.7918, -139.6875) (-124.9621, -139.2197) (-125.5712, -138.8287) (-126.1453, -138.8187) knots 0 0 0 0 1 1 1 1
  spline S40 degree 3 poles (-126.1453, -138.8187) (-126.7195, -138.8087) (-127.4424, -138.105) (-127.7519, -137.2548) knots 0 0 0 0 1 1 1 1
  spline S41 degree 3 poles (-127.7519, -137.2548) (-128.1329, -136.2081) (-128.6652, -135.819) (-129.4007, -136.0498) knots 0 0 0 0 1 1 1 1
  spline S42 degree 3 poles (-129.4007, -136.0498) (-130.085, -136.2645) (-129.9482, -135.9374) (-129.0308, -135.166) knots 0 0 0 0 1 1 1 1
  spline S43 degree 3 poles (-129.0308, -135.166) (-127.3423, -133.7459) (-127.582, -132.679) (-130.5025, -128.6131) knots 0 0 0 0 1 1 1 1
  spline S44 degree 3 poles (-130.5025, -128.6131) (-135.3605, -121.8502) (-135.4133, -121.7401) (-135.9917, -117.1824) knots 0 0 0 0 1 1 1 1
  spline S45 degree 3 poles (-135.9917, -117.1824) (-136.2994, -114.7575) (-137.1556, -110.6593) (-137.8943, -108.0755) knots 0 0 0 0 1 1 1 1
  spline S46 degree 3 poles (-137.8943, -108.0755) (-138.633, -105.4917) (-139.1612, -102.8242) (-139.0681, -102.1478) knots 0 0 0 0 1 1 1 1
  spline S47 degree 3 poles (-139.0681, -102.1478) (-138.9659, -101.4044) (-139.1827, -100.8591) (-139.6164, -100.7692) knots 0 0 0 0 1 1 1 1
  spline S48 degree 3 poles (-139.6164, -100.7692) (-140.0109, -100.6874) (-140.326, -100.1727) (-140.3165, -99.6255) knots 0 0 0 0 1 1 1 1
  spline S49 degree 3 poles (-140.3165, -99.6255) (-140.307, -99.0782) (-141.0618, -97.9071) (-141.9939, -97.0229) knots 0 0 0 0 1 1 1 1
  spline S50 degree 3 poles (-141.9939, -97.0229) (-142.926, -96.1388) (-144.4149, -93.9458) (-145.3026, -92.1497) knots 0 0 0 0 1 1 1 1
  spline S51 degree 3 poles (-145.3026, -92.1497) (-146.1903, -90.3535) (-147.6639, -88.2222) (-148.5772, -87.4136) knots 0 0 0 0 1 1 1 1
  spline S52 degree 3 poles (-148.5772, -87.4136) (-149.6517, -86.4623) (-150.5685, -84.8339) (-151.1746, -82.8005) knots 0 0 0 0 1 1 1 1
  line L91 (-151.1746, -82.8005) -> (-152.1113, -79.6578)
  line L92 (-152.1113, -79.6578) -> (-145.0725, -76.8727)
  line L93 (-145.0725, -76.8727) -> (-139.6588, -79.8807)
  line L94 (-139.6588, -79.8807) -> (-139.6591, -79.8813)
  spline S53 degree 3 poles (-139.6591, -79.8813) (-136.6816, -81.5357) (-133.4883, -83.6932) (-132.5628, -84.676) knots 0 0 0 0 1 1 1 1
  spline S54 degree 3 poles (-132.5628, -84.676) (-130.6273, -86.7309) (-125.8288, -89.0335) (-121.5387, -89.9657) knots 0 0 0 0 1 1 1 1
  line L95 (-121.5387, -89.9657) -> (-118.5791, -90.609)
  line L96 (-118.5791, -90.609) -> (-116.5906, -88.5651)
  spline S55 degree 3 poles (-116.5906, -88.5651) (-114.2332, -86.142) (-111.3799, -79.5261) (-109.9199, -73.0985) knots 0 0 0 0 1 1 1 1
  spline S56 degree 3 poles (-109.9199, -73.0985) (-108.891, -68.5684) (-108.2546, -67.383) (-107.6608, -68.8907) knots 0 0 0 0 1 1 1 1
  spline S57 degree 3 poles (-107.6608, -68.8907) (-107.497, -69.3066) (-106.4548, -71.4025) (-105.3449, -73.5484) knots 0 0 0 0 1 1 1 1
  spline S58 degree 3 poles (-105.3449, -73.5484) (-103.5984, -76.9253) (-103.3705, -77.8432) (-103.6508, -80.373) knots 0 0 0 0 1 1 1 1
  spline S59 degree 3 poles (-128.3872, -72.8102) (-129.4627, -71.613) (-134.1338, -70.2563) (-133.2081, -68.992) knots 0 0 0 0 1 1 1 1
  spline S60 degree 3 poles (-133.2081, -68.992) (-131.2389, -68.4482) (-130.936, -67.0047) (-129.6791, -65.9357) knots 0 0 0 0 1 1 1 1
  spline S61 degree 3 poles (-129.6791, -65.9357) (-125.8343, -62.6694) (-127.4522, -73.1016) (-127.616, -73.2152) knots 0 0 0 0 1 1 1 1
  line L97 (-127.616, -73.2152) -> (-127.616, -73.215)
  spline S62 degree 3 poles (-127.616, -73.215) (-127.919, -73.3253) (-128.2661, -73.1431) (-128.3872, -72.8102) knots 0 0 0 0 1 1 1 1
  spline S63 degree 3 poles (-323.6954, -82.9764) (-325.8373, -84.9793) (-332.4297, -89.2945) (-338.345, -92.5656) knots -1 -1 -1 -1 0 0 0 0
  spline S64 degree 3 poles (-338.345, -92.5656) (-344.2602, -95.8368) (-349.7543, -99.04) (-350.5537, -99.6841) knots -1 -1 -1 -1 0 0 0 0
  spline S65 degree 3 poles (-350.5537, -99.6841) (-354.1072, -102.5467) (-355.0753, -99.9681) (-355.0753, -87.6398) knots -1 -1 -1 -1 0 0 0 0
  spline S66 degree 3 poles (-355.0753, -87.6398) (-355.0753, -73.0985) (-355.8141, -72.1224) (-363.9321, -75.9411) knots -1 -1 -1 -1 0 0 0 0
  spline S67 degree 3 poles (-363.9321, -75.9411) (-366.9481, -77.36) (-369.595, -78.9241) (-369.8141, -79.4171) knots -1 -1 -1 -1 0 0 0 0
  spline S68 degree 3 poles (-369.8141, -79.4171) (-370.4737, -80.9013) (-373.5893, -80.4246) (-373.7194, -78.8195) knots -1 -1 -1 -1 0 0 0 0
  spline S69 degree 3 poles (-373.7194, -78.8195) (-374.5603, -68.447) (-369.832, -61.6467) (-365.0199, -66.3073) knots -1 -1 -1 -1 0 0 0 0
  spline S70 degree 3 poles (-365.0199, -66.3073) (-362.7421, -68.5136) (-347.5821, -75.5333) (-345.0961, -75.5333) knots -1 -1 -1 -1 0 0 0 0
  spline S71 degree 3 poles (-345.0961, -75.5333) (-343.9388, -75.5333) (-341.2628, -74.2576) (-339.1495, -72.6985) knots -1 -1 -1 -1 0 0 0 0
  spline S72 degree 3 poles (-339.1495, -72.6985) (-337.0362, -71.1394) (-332.7639, -68.9128) (-329.6558, -67.7504) knots -1 -1 -1 -1 0 0 0 0
  spline S73 degree 3 poles (-329.6558, -67.7504) (-326.5477, -66.5881) (-323.4669, -65.2358) (-322.8096, -64.7452) knots -1 -1 -1 -1 0 0 0 0
  line L98 (-322.8096, -64.7452) -> (-322.8094, -64.7455)
  spline S74 degree 3 poles (-322.8094, -64.7455) (-322.1521, -64.2549) (-319.4481, -63.4967) (-316.8004, -63.0606) knots -1 -1 -1 -1 0 0 0 0
  spline S75 degree 3 poles (-316.8004, -63.0606) (-312.7018, -62.3855) (-311.5923, -62.6875) (-309.3317, -65.0938) knots -1 -1 -1 -1 0 0 0 0
  spline S76 degree 3 poles (-309.3317, -65.0938) (-305.2318, -69.4575) (-306.0084, -71.5505) (-313.2386, -75.6312) knots -1 -1 -1 -1 0 0 0 0
  spline S77 degree 3 poles (-313.2386, -75.6312) (-316.8479, -77.6681) (-321.5535, -80.9736) (-323.6954, -82.9764) knots -1 -1 -1 -1 0 0 0 0
  line L99 (-76.8192, -215.9) -> (-79.4365, -211.2784)
  spline S78 degree 3 poles (-79.4365, -211.2784) (-81.2221, -208.1253) (-83.5633, -204.6981) (-84.6389, -203.663) knots 0 0 0 0 1 1 1 1
  spline S79 degree 3 poles (-84.6389, -203.663) (-86.6971, -201.6816) (-90.5134, -195.9478) (-89.9214, -195.7261) knots 0 0 0 0 1 1 1 1
  spline S80 degree 3 poles (-89.9214, -195.7261) (-89.7309, -195.6547) (-90.4659, -193.0438) (-91.5548, -189.9237) knots 0 0 0 0 1 1 1 1
  spline S81 degree 3 poles (-91.5548, -189.9237) (-92.8333, -186.2605) (-93.4883, -183.3011) (-93.4037, -181.5704) knots 0 0 0 0 1 1 1 1
  spline S82 degree 3 poles (-93.4037, -181.5704) (-93.2975, -179.3971) (-93.9219, -177.2686) (-96.7029, -170.3232) knots 0 0 0 0 1 1 1 1
  spline S83 degree 3 poles (-96.7029, -170.3232) (-100.0171, -162.0462) (-100.2006, -161.7333) (-102.1257, -161.073) knots 0 0 0 0 1 1 1 1
  spline S84 degree 3 poles (-102.1257, -161.073) (-103.2216, -160.6969) (-104.2696, -159.9735) (-104.4545, -159.4656) knots 0 0 0 0 1 1 1 1
  spline S85 degree 3 poles (-104.4545, -159.4656) (-104.6393, -158.9576) (-105.2292, -158.3375) (-105.7651, -158.0876) knots 0 0 0 0 1 1 1 1